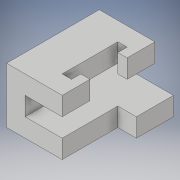
# Autodesk Inventor part: P3-7
Saved by Autodesk Inventor 2017 (Build 210142000, 142)
## iProperties
Created: 2017-02-12
Part Number: P3-7
Material: Generic
Document SubType Name: Modeling
Designer: Schaffel
Density: 1 g/cm^3
Appearance: Default
Author: Schaffel
Autodesk Inventor part; units mm, degrees
ref_plane "YZ Plane" through (0, 0, 0) normal (1, 0, 0) x (0, 1, 0)
ref_plane "XZ Plane" through (0, 0, 0) normal (0, 1, 0) x (-1, 0, 0)
ref_plane "XY Plane" through (0, 0, 0) normal (0, 0, 1) x (1, 0, 0)
sketch "Sketch1" plane through (0, 0, 0) normal (0, 0, 1) x (1, 0, 0)
  point P0 (0, 0)
sketch "Sketch2" plane through (0, 0, 0) normal (0, 0, 1) x (1, 0, 0)
  line L0 (0, 0) -> (50.8, 0)
  line L1 (50.8, 0) -> (50.8, 12.7)
  line L2 (50.8, 12.7) -> (12.7, 12.7)
  line L3 (12.7, 12.7) -> (12.7, 25.4)
  line L4 (12.7, 25.4) -> (38.1, 25.4)
  line L5 (38.1, 25.4) -> (38.1, 38.1)
  line L6 (38.1, 38.1) -> (0, 38.1)
  line L7 (0, 38.1) -> (0, 0)
  constraints: 16 end point, 7 perpendicular
extrude "Extrusion1" add sketch "Sketch2" along normal blind 63.5
sketch "Sketch3" plane through (12.7, 12.7, 0) normal (0, 1, 0) x (1, 0, 0)
  line L0 (38.1, -25.4) -> (25.4, -25.4)
  line L1 (25.4, -25.4) -> (25.4, -63.5)
  line L2 (38.1, -63.5) -> (0, -63.5) projected
  line L3 (25.4, -63.5) -> (38.1, -63.5)
  line L4 (38.1, -63.5) -> (38.1, -25.4)
  point P0 (-12.7, 0)
  constraints: 8 end point, 2 perpendicular, 1 collinear, 1 point on line
extrude "Extrusion2" cut sketch "Sketch3" against normal blind 12.7
sketch "Sketch4" plane through (0, 38.1, 0) normal (0, 1, 0) x (1, 0, 0)
  line L0 (38.1, 0) -> (38.1, -63.5) projected
  line L1 (38.1, -19.05) -> (31.75, -19.05)
  line L2 (31.75, -19.05) -> (31.75, -12.7)
  line L3 (31.75, -12.7) -> (25.4, -12.7)
  line L4 (25.4, -12.7) -> (25.4, -50.8)
  line L5 (25.4, -50.8) -> (31.75, -50.8)
  line L6 (31.75, -50.8) -> (31.75, -44.45)
  line L7 (31.75, -44.45) -> (38.1, -44.45)
  line L8 (38.1, -44.45) -> (38.1, -19.05)
  point P0 (0, 0)
  constraints: 16 end point, 4 perpendicular, 2 point on line
extrude "Extrusion3" cut sketch "Sketch4" against normal blind 12.7
body "Solid1"
